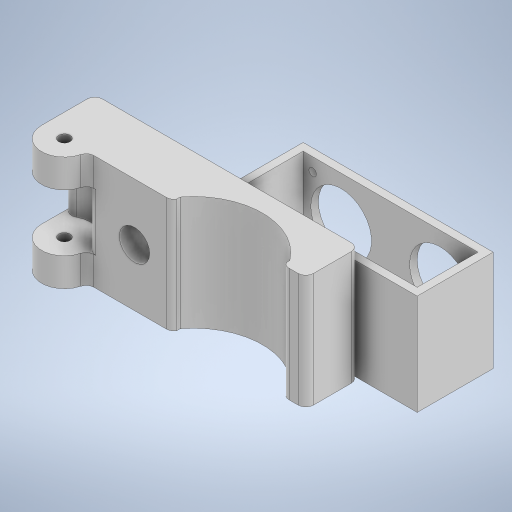
# Autodesk Inventor part: Bike_Mount_Right
Saved by Autodesk Inventor 2023 (Build 270158000, 158)
## iProperties
Created: 2023-01-23
Part Number: Bike_Mount_Right
Material: Generic
Document SubType Name: Modeling
Designer: manny
Density: 1 g/cm^3
Appearance: Default
Author: manny
Autodesk Inventor part; units mm, degrees
ref_plane "YZ Plane" through (0, 0, 0) normal (1, 0, 0) x (0, 1, 0)
ref_plane "XZ Plane" through (0, 0, 0) normal (0, 1, 0) x (-1, 0, 0)
ref_plane "XY Plane" through (0, 0, 0) normal (0, 0, 1) x (1, 0, 0)
sketch "Sketch2" plane through (0, 0, 0) normal (0, 1, 0) x (-1, 0, 0)
  line L0 (3.9324, 0) -> (5, 0)
  arc A0 (3.9324, 0) -> (1.9324, -2) centre (3.9324, -2) ccw
  line L1 (3.9324, 0) -> (6.9065, 0)
  line L2 (3.9324, 0) -> (6.3389, 0)
  arc A1 (7.9907, -0.8725) -> (36.874, -0.8725) centre (22.4324, 8.9853) ccw
  line L3 (38.5258, 0) -> (57.6864, 0)
  arc A2 (71.4324, 0) -> (59.6229, 1.5) centre (65.4324, 0) ccw
  circle A3 centre (65.4324, 0) radius 1.5
  arc A4 (57.6864, 0) -> (59.6229, 1.5) centre (57.6864, 2) ccw
  arc A5 (38.5258, 0) -> (36.874, -0.8725) centre (38.5258, -2) ccw
  arc A6 (7.9907, -0.8725) -> (6.3389, 0) centre (6.3389, -2) ccw
  arc A7 (59.3504, -1.7983) -> (57.1879, 0) centre (57.1879, -2.1995) ccw
  line L4 (77.1831, 8.9853) -> (-10.6505, 8.9853) construction
  line L5 (3.9324, 17.9706) -> (5, 17.9706)
  arc A8 (42.998, 40.9699) -> (1.9324, 19.9706) centre (55.0831, -33.3161) ccw
  arc A9 (1.9324, 19.9706) -> (3.9324, 17.9706) centre (3.9324, 19.9706) ccw
  line L6 (3.9324, 17.9706) -> (6.9065, 17.9706)
  line L7 (3.9324, 17.9706) -> (6.3389, 17.9706)
  arc A10 (36.874, 18.843) -> (7.9907, 18.843) centre (22.4324, 8.9853) ccw
  line L8 (38.5258, 17.9706) -> (57.6864, 17.9706)
  arc A11 (59.6229, 16.4706) -> (71.4324, 17.9706) centre (65.4324, 17.9706) ccw
  arc A12 (71.4324, 17.9706) -> (42.998, 40.9699) centre (43.4479, 12.4496) ccw
  circle A13 centre (65.4324, 17.9706) radius 1.5
  arc A14 (59.6229, 16.4706) -> (57.6864, 17.9706) centre (57.6864, 15.9706) ccw
  arc A15 (36.874, 18.843) -> (38.5258, 17.9706) centre (38.5258, 19.9706) ccw
  arc A16 (6.3389, 17.9706) -> (7.9907, 18.843) centre (6.3389, 19.9706) ccw
  arc A17 (65.6797, 24.421) -> (59.3504, 19.7689) centre (64.5387, 19.3419) ccw
  arc A18 (65.6797, 24.421) -> (67.6049, 27.617) centre (65.5936, 26.6507) ccw
  arc A19 (57.1879, 17.9706) -> (59.3504, 19.7689) centre (57.1879, 20.1701) ccw
  line L9 (1.9324, -2) -> (1.9324, -12)
  line L10 (3.9324, -14) -> (69.4324, -14)
  arc A20 (1.9324, -12) -> (3.9324, -14) centre (3.9324, -12) ccw
  line L11 (71.4324, 0) -> (71.4324, -12)
  arc A21 (69.4324, -14) -> (71.4324, -12) centre (69.4324, -12) ccw
  arc A22 (59.3504, -1.7983) -> (71.4324, -2.4583) centre (65.4715, -0.6626) ccw
  point P0 (0, 0)
  point P1 (7.4324, 0)
  point P2 (37.4324, 0)
  point P3 (22.4324, -8.5)
  point P4 (0, 17.9706)
  point P5 (7.4324, 17.9706)
  point P6 (37.4324, 17.9706)
  point P7 (22.4324, 26.4706)
  point P8 (71.4324, 17.9706)
  point P9 (6.3389, 17.9706)
  dimension "d3" = 2
  dimension "d12" = 3.5
  dimension "d13" = 30
  dimension "d14" = 8.5
  dimension "d17" = 3
  dimension "d18" = 2
  dimension "d19" = 2
  dimension "d21" = 0
  dimension "d22" = 0
  dimension "d91" = 3.9324
  dimension "d92" = 2
  dimension "d93" = 28
  dimension "d94" = 2
  dimension "d107" = 10
  constraints: 51 point on circle, 25 symmetric about line, 24 end point, 23 centre point, 15 tangent, 11 point on line, 5 horizontal, 2 coincident, 2 vertical, 1 equal radius, 8 other
  measures "d3" radius of A0
  measures "d12" distance of L0.start point (7.432, 0)
  measures "d13" distance of point (7.432, 0) point (37.432, 0)
  measures "d14" vertical distance of point (7.432, 0) point (22.432, -8.5)
  measures "d17" diameter of A3
  measures "d18" radius of A4
  measures "d19" radius of A6
  measures "d21" vertical distance of point (0, 0) A2.centre
  measures "d22" distance from line of point (0, 0) L3
  measures "d91" distance of L0.start point (0, 0)
  measures "d92" radius of A20
  measures "d93" distance of A2.centre point (37.432, 0)
  measures "d94" radius of A21
  measures "d107" distance of L9.start L9.end
extrude "Extrusion1" add sketch "Sketch2" along normal mid plane 30 contours L0 L1 A6 A1 A5 L3 A7 A22 L11 A21 L10 A20 L9 A0 | L3 A4 A2 L11 A22 A7
extrude "Extrusion2" cut sketch "Sketch2" along normal mid plane 15 contours L3 A4 A2 L11 A22 A7
sketch "Sketch7" plane through (0, -15, 0) normal (0, -1, 0) x (1, 0, 0)
  arc A0 (-6.3389, 0) -> (-7.9907, -0.8725) centre (-6.3389, -2) ccw projected
  line L0 (-7.9907, -0.8725) -> (-7.9907, -1.8725)
  arc A1 (-36.874, -0.8725) -> (-7.9907, -0.8725) centre (-22.4324, 8.9853) ccw projected
  line L1 (-36.874, -0.8725) -> (-36.874, -1.8725)
  arc A2 (-36.874, -1.8725) -> (-7.9907, -1.8725) centre (-22.4324, 8.9853) ccw
  point P0 (0, 0)
  dimension "d59" = 1
  dimension "d60" = 1
  constraints: 4 end point, 2 point on circle, 2 vertical, 1 centre point
  measures "d59" distance of L0.start L0.end
  measures "d60" distance of L1.start L1.end
extrude "Extrusion10" cut sketch "Sketch7" against normal up to next
fillet "Fillet4" radius 2 1 edges at (-71.4324, 0, -2.4583)
sketch "Sketch13" plane through (-57.6864, -15, 0) normal (0, 0, 1) x (1, 0, 0)
  circle A0 centre (10.6864, 15) radius 4
  line L0 (55.754, 30) -> (55.754, 0) projected
  point P0 (57.6864, 15)
  dimension "d99" = 8
  dimension "d106" = 47
  constraints: 1 centre point
  measures "d99" diameter of A0
  measures "d106" distance of A0.centre point (57.686, 15)
extrude "Extrusion15" cut sketch "Sketch13" against normal up to next
sketch "Sketch14" plane through (-3.9324, 15, -14) normal (0, 0, -1) x (-1, 0, 0)
  circle A0 centre (43.0676, -15) radius 4 projected
  line L0 (43.0676, -21.3509) -> (37.5676, -18.1754)
  line L1 (37.5676, -18.1754) -> (37.5676, -11.8246)
  line L2 (37.5676, -11.8246) -> (43.0676, -8.6491)
  line L3 (43.0676, -8.6491) -> (48.5676, -11.8246)
  line L4 (48.5676, -11.8246) -> (48.5676, -18.1754)
  line L5 (48.5676, -18.1754) -> (43.0676, -21.3509)
  line L6 (67.5, -30) -> (67.5, 0) projected
  point P0 (-3.9324, -15)
  point P1 (37.5676, -15)
  dimension "d103" = 11
  constraints: 12 end point, 1 coincident, 1 midpoint, 1 parallel, 13 other
  measures "d103" distance from line of point (37.568, -15) L4
extrude "Extrusion16" cut sketch "Sketch14" against normal blind 2
sketch "Sketch15" plane through (-3.9324, 15, -14) normal (0, 0, -1) x (-1, 0, 0)
  line L0 (32.6944, -26.5) -> (-17.3056, -26.5)
  line L1 (-17.3056, -26.5) -> (-17.3056, -3.5)
  line L2 (-17.3056, -3.5) -> (32.6944, -3.5)
  line L3 (32.6944, -3.5) -> (32.6944, -26.5)
  line L4 (0, 0) -> (65.5, 0) projected
  line L5 (32.9416, -30) -> (4.0584, -30) projected
  line L6 (-17.3056, -26.5) -> (32.75, -26.5)
  line L7 (32.75, -26.5) -> (32.75, -30)
  line L8 (32.75, -30) -> (-17.3056, -30)
  line L9 (-17.3056, -30) -> (-17.3056, -26.5)
  point P0 (7.6944, -26.5)
  point P1 (4.0584, -30)
  dimension "d111" = 50
  dimension "d112" = 23
  constraints: 16 end point, 4 parallel, 2 horizontal, 2 perpendicular, 1 midpoint, 1 point on line
  measures "d111" distance of L1.end L2.end
  measures "d112" distance of L0.end L1.end
extrude "Extrusion17" add sketch "Sketch15" along normal blind 20
sketch "Sketch17" plane through (-3.9324, 15, -34) normal (0, 0, -1) x (-1, 0, 0)
  line L0 (-17.3056, -26.5) -> (32.75, -26.5)
  line L1 (32.75, -30) -> (-17.3056, -30)
  line L2 (32.6944, -26.5) -> (-17.3056, -26.5)
  line L3 (-17.3056, -3.5) -> (32.6944, -3.5)
  circle A0 centre (-12.8056, -23.5) radius 1
  line L4 (-17.3056, -26.5) -> (-17.3056, -3.5)
  line L5 (-17.3056, -30) -> (-17.3056, -26.5)
  circle A1 centre (-5.3045, -15.2368) radius 8
  circle A2 centre (20.6944, -15) radius 8
  line L6 (32.75, -26.5) -> (32.75, -30)
  line L7 (32.9416, -30) -> (4.0584, -30)
  line L8 (32.6944, -3.5) -> (32.6944, -26.5)
  circle A3 centre (28.1944, -7) radius 1
  point P0 (-3.9324, -15)
  point P1 (-3.9324, -15)
  point P2 (7.6944, -26.5)
  point P3 (-3.9324, -15)
  point P4 (0, 0)
  point P5 (7.6944, -13.0925)
  dimension "d142" = 50
  dimension "d143" = 23
  dimension "d144" = 25
  dimension "d145" = 2
  dimension "d146" = 2
  dimension "d147" = 41
  dimension "d148" = 16.5
  dimension "d149" = 3.5
  dimension "d150" = 4.5
  dimension "d151" = 16
  dimension "d152" = 16
  dimension "d153" = 26
  dimension "d154" = 11.5
  dimension "d155" = 13
  constraints: 18 end point, 4 centre point, 4 parallel, 2 horizontal, 2 perpendicular, 1 midpoint, 1 point on line
  measures "d142" distance of L3.start L8.start
  measures "d143" distance of L0.start L3.start
  measures "d144" distance from line of L4 point (7.694, -13.093)
  measures "d145" diameter of A3
  measures "d146" diameter of A0
  measures "d147" horizontal distance of A0.centre A3.centre
  measures "d148" vertical distance of A3.centre A0.centre
  measures "d149" distance from line of L3 A3.centre
  measures "d150" distance from line of L8 A3.centre
  measures "d151" diameter of A2
  measures "d152" diameter of A1
  measures "d153" distance of A1.centre A2.centre
  measures "d154" distance from line of L2 A2.centre
  measures "d155" horizontal distance of point (7.694, -13.093) A2.centre
extrude "Extrusion18" cut sketch "Sketch17" against normal blind 2 contours A0 | A1 | A2 | A3
sketch "Sketch18" plane through (-3.9324, 11.5, -14) normal (0, 1, 0) x (1, 0, 0)
  line L0 (-30.6944, 2) -> (15.3056, 2)
  line L1 (15.3056, 2) -> (15.3056, 18)
  line L2 (15.3056, 18) -> (-30.6944, 18)
  line L3 (-30.6944, 18) -> (-30.6944, 2)
  line L4 (-32.6944, 20) -> (17.3056, 20) projected
  line L5 (0, 0) -> (-65.5, 0) projected
  line L6 (17.3056, 0) -> (17.3056, 20) projected
  line L7 (-32.6944, 0) -> (-32.6944, 20) projected
  point P0 (3.9324, -14)
  dimension "d158" = 2
  dimension "d159" = 2
  dimension "d160" = 2
  dimension "d161" = 2
  constraints: 8 end point, 2 parallel, 1 horizontal, 1 perpendicular
  measures "d158" distance between parallel lines of L4 L2
  measures "d159" distance between parallel lines of L5 L0
  measures "d160" distance between parallel lines of L6 L1
  measures "d161" distance between parallel lines of L7 L3
extrude "Extrusion19" cut sketch "Sketch18" against normal blind 21
sketch "Sketch19" plane through (-3.9324, -9.5, -14) normal (0, 1, 0) x (1, 0, 0)
  line L0 (-30.6944, 18) -> (12.8056, 18) projected
  line L1 (-15.6944, 6) -> (0.3056, 6)
  line L2 (0.3056, 6) -> (0.3056, 18)
  line L3 (0.3056, 18) -> (-15.6944, 18)
  line L4 (-15.6944, 18) -> (-15.6944, 6)
  line L5 (-30.6944, 2) -> (-30.6944, 18) projected
  point P0 (3.9324, -14)
  point P1 (-15.6944, 18)
  dimension "d164" = 15
  dimension "d165" = 16
  dimension "d168" = 12
  constraints: 8 end point, 2 parallel, 1 horizontal, 1 perpendicular, 1 point on line
  measures "d164" distance between parallel lines of L5 L4
  measures "d165" distance between parallel lines of L2 L4
  measures "d168" distance of L3.end L1.start
extrude "Extrusion20" cut sketch "Sketch19" against normal blind 20
body "Solid1"
